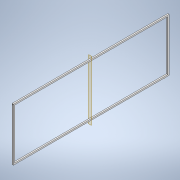
# Autodesk Inventor part: porta1
Saved by Autodesk Inventor 2022 (Build 260153000, 153)
## iProperties
Created: 2022-08-29
Part Number: porta1
Material: Generic
Document SubType Name: Modeling
Designer: cvss2
Density: 1 g/cm^3
Appearance: Default
Author: cvss2
Autodesk Inventor part; units mm, degrees
ref_plane "YZ Plane" through (0, 0, 0) normal (1, 0, 0) x (0, 1, 0)
ref_plane "XZ Plane" through (0, 0, 0) normal (0, 1, 0) x (-1, 0, 0)
ref_plane "XY Plane" through (0, 0, 0) normal (0, 0, 1) x (1, 0, 0)
sketch "Sketch1" plane through (0, 0, 0) normal (1, 0, 0) x (0, 1, 0)
  line L0 (0, 0) -> (-383, 0)
  line L1 (-383, 0) -> (-383, -1138)
  line L2 (-383, -1138) -> (0, -1138)
  line L3 (0, -1138) -> (0, 0)
  line L4 (-373, -1128) -> (-373, -10)
  line L5 (-373, -10) -> (-10, -10)
  line L6 (-10, -10) -> (-10, -1128)
  line L7 (-10, -1128) -> (-373, -1128)
  dimension "d0" = 383
  dimension "d1" = 1138
  dimension "d2" = 10
  constraints: 16 end point, 4 parallel, 2 perpendicular, 1 horizontal, 3 other
  measures "d0" distance of L2.end L1.end
  measures "d1" distance of L1.end L0.end
  measures "d2" distance between parallel lines of L1 L4
extrude "Extrusion1" add sketch "Sketch1" along normal blind 10
sketch "Sketch2" plane through (0, -383, 0) normal (0, 0, 1) x (1, 0, 0)
  line L0 (0, 383) -> (0, 0) projected
  line L1 (0, 0) -> (10, 0) projected
  line L2 (10, 383) -> (10, 0) projected
  line L3 (0, 383) -> (10, 383) projected
  line L4 (0, 0) -> (-3.182, -3.182)
  line L5 (0, 0) -> (4.5, 0) construction
  line L6 (0, 383) -> (0, 0) projected
  circle A0 centre (-3.182, -3.182) radius 5
  circle A1 centre (-3.182, -3.182) radius 4
  dimension "d5" = 4.5
  dimension "d6" = 135
  dimension "d7" = 1
  dimension "d10" = 10
  constraints: 4 end point, 2 centre point, 1 coincident, 1 equal length, 1 horizontal
  measures "d5" distance of L0.end L4.end
  measures "d6" angle of L4 L5
  measures "d7" radial gap between concentric circles of A0 A1
  measures "d10" diameter of A0
extrude "Extrusion2" add sketch "Sketch2" against normal blind 35 contours A0 L1 L0 | L0 L1 A0
ref_plane "Work Plane1" through (0, 0, -569) normal (0, 0, 1) x (1, 0, 0)
mirror "Mirror1" about plane through (0, 0, -569) normal (0, 0, 1) of "Extrusion2"
fillet "Fillet1" [suppressed]
ref_plane "Work Plane2" through (0, -383, -1113) normal (0, 0, 1) x (1, 0, 0)
sketch "Sketch3" plane through (0, -383, -1113) normal (0, 0, 1) x (1, 0, 0)
  arc A0 (0, 0.6748) -> (0.6748, 0) centre (-3.182, -3.182) ccw projected
  circle A1 centre (-3.182, -3.182) radius 4 projected
  line L0 (0.6748, 0) -> (10, 0) projected
  circle A2 centre (-3.182, -3.182) radius 5
  point P0 (0, 383)
  point P1 (0, 0.6748)
  constraints: 1 coincident, 3 other
extrude "Extrusion3" cut sketch "Sketch3" against normal blind 15
sketch "Sketch4" plane through (0, 0, 0) normal (0, 0, 1) x (1, 0, 0)
  circle A0 centre (-3.182, -386.182) radius 4 projected
  arc A1 (0, -382.3252) -> (0.6748, -383) centre (-3.182, -386.182) ccw projected
  circle A2 centre (-3.182, -386.182) radius 4 projected
  line L0 (0.6748, -383) -> (10, -383) projected
  circle A3 centre (-3.182, -386.182) radius 5
  point P0 (0, 0)
  point P1 (0, -382.3252)
  constraints: 1 coincident, 3 other
extrude "Extrusion4" cut sketch "Sketch4" against normal blind 10
sketch "Sketch5" plane through (0, -383, -35) normal (0, 0, -1) x (-1, 0, 0)
  circle A0 centre (3.182, -3.182) radius 4 projected
  arc A1 (-0.6748, 0) -> (0, 0.6748) centre (3.182, -3.182) ccw projected
  circle A2 centre (3.182, -3.182) radius 5
  point P0 (0, 383)
  point P1 (0, 0.6748)
  constraints: 1 coincident, 3 other
extrude "Extrusion5" cut sketch "Sketch5" against normal blind 10
sketch "Sketch6" plane through (0, 0, 0) normal (0, 0, 1) x (1, 0, 0)
  arc A0 (0.6748, -383) -> (0, -382.3252) centre (-3.182, -386.182) ccw projected
  line L0 (0.6748, -383) -> (10, -383) projected
  line L1 (10, 0) -> (10, -383) projected
  line L2 (0, 0) -> (10, 0) projected
  line L3 (0, 0) -> (0, -382.3252) projected
  line L4 (10, -383) -> (10, 0) construction
  line L5 (0, -10) -> (10, -10) construction
  line L6 (10, 0) -> (0, -10) construction
  line L7 (0, 0) -> (10, 0) construction
  line L8 (0, 0) -> (10, -10) construction
  circle A1 centre (5, -5) radius 2.5
  dimension "d19" = 5
  constraints: 4 end point, 1 centre point, 1 midpoint
  measures "d19" diameter of A1
extrude "Extrusion6" cut sketch "Sketch6" against normal blind 3 contours A1
sketch "Sketch7" plane through (5, -5, -3) normal (0, 0, 1) x (1, 0, 0)
  circle A0 centre (0, 0) radius 2.5 projected
  circle A1 centre (0, 0) radius 7.5
  line L0 (13, -13) -> (-13, -13)
  line L1 (-13, -13) -> (-13, 13)
  line L2 (-13, 13) -> (13, 13)
  line L3 (13, 13) -> (13, -13)
  line L4 (13, -13) -> (-13, 13) construction
  line L5 (-13, -13) -> (13, 13) construction
  point P0 (-5, 5)
  dimension "d22" = 15
  dimension "d25" = 26
  dimension "d26" = 26
  constraints: 12 end point, 2 midpoint, 2 parallel, 1 centre point, 1 coincident, 1 horizontal, 1 perpendicular
  measures "d22" diameter of A1
  measures "d25" distance of L1.end L2.end
  measures "d26" distance of L0.end L1.end
extrude "Extrusion7" [suppressed]
mirror "Mirror2" about plane through (0, 0, -569) normal (0, 0, 1) of "Extrusion6"
equation "\"d25\" = d26"
body "Solid1"
